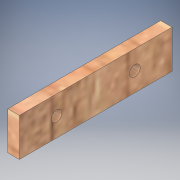
# Autodesk Inventor part: КВ33.044.406 - Прижим ремня
Saved by Autodesk Inventor 2019 (Build 230136000, 136)
## iProperties
Created: 2019-08-20
Part Number: КВ33.044.406 - Прижим ремня
Material: Дерево (береза)
Document SubType Name: Modeling
Designer: Петров Иван
Density: 0.55 g/cm^3
Appearance: Береза — натуральный — полированный
Author: Петров Иван
Autodesk Inventor part; units mm, degrees
ref_plane "YZ Plane" through (0, 0, 0) normal (1, 0, 0) x (0, 1, 0)
ref_plane "XZ Plane" through (0, 0, 0) normal (0, 1, 0) x (-1, 0, 0)
ref_plane "XY Plane" through (0, 0, 0) normal (0, 0, 1) x (1, 0, 0)
sketch "Эскиз1" plane through (0, 0, 0) normal (1, 0, 0) x (0, 1, 0)
  line L0 (-5, 20) -> (5, 20)
  line L1 (5, 20) -> (5, -20)
  line L2 (5, -20) -> (-5, -20)
  line L3 (-5, -20) -> (-5, 20)
  line L4 (0, 0) -> (0, 10.236)
  line L5 (0, 0) -> (0, -10.236)
  circle A0 centre (0, 10.236) radius 1.4
  circle A1 centre (0, -10.236) radius 1.4
  dimension "d0" = 10
  dimension "d1" = 40
  dimension "d10" = 10.236
  dimension "d11" = 10.236
  dimension "d12" = 2.8
  dimension "d13" = 2.8
  constraints: 12 end point, 2 centre point, 2 coincident, 2 parallel, 2 vertical, 1 horizontal, 1 perpendicular
  measures "d0" distance of L1.end L2.end
  measures "d1" distance of L0.end L1.end
  measures "d10" distance of L4.start L4.end
  measures "d11" distance of L4.start L5.end
  measures "d12" diameter of A0
  measures "d13" diameter of A1
extrude "Выдавливание1" add sketch "Эскиз1" along normal blind 3
equation "\"d11\" = d10"
